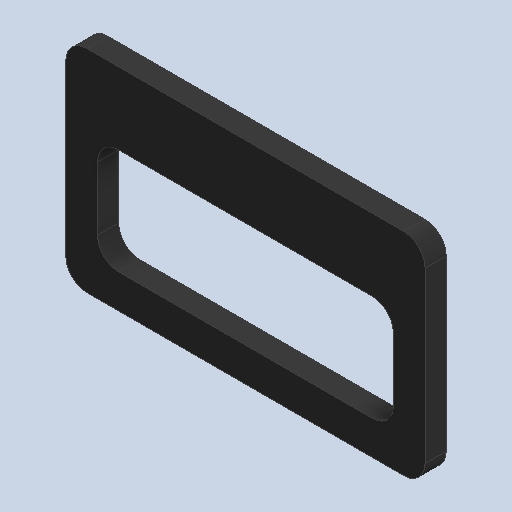
# Autodesk Inventor part: CAMERA_CON_SPACER
Saved by Autodesk Inventor 2024.2 (Build 282272000, 272)
## iProperties
Created: 2020-06-21
Part Number: CAMERA_CON_SPACER
Material: Generic
Document SubType Name: Modeling
Designer: Viktor Lindström
Density: 1 g/cm^3
Appearance: Default
Author: Viktor Lindström
Autodesk Inventor part; units mm, degrees
ref_plane "YZ Plane" through (0, 0, 0) normal (1, 0, 0) x (0, 1, 0)
ref_plane "XZ Plane" through (0, 0, 0) normal (0, 1, 0) x (-1, 0, 0)
ref_plane "XY Plane" through (0, 0, 0) normal (0, 0, 1) x (1, 0, 0)
sketch "Sketch1" plane through (0, 0, 0) normal (0, 0, 1) x (1, 0, 0)
  line L0 (-8.5, -5) -> (8.5, -5)
  line L1 (8.5, -5) -> (8.5, 5)
  line L2 (8.5, 5) -> (-8.5, 5)
  line L3 (-8.5, 5) -> (-8.5, -5)
  line L4 (-8.5, -5) -> (8.5, 5) construction
  line L5 (8.5, -5) -> (-8.5, 5) construction
  line L6 (0, -7) -> (0, 7) construction
  line L7 (-7, -3.4) -> (7, -3.4)
  line L8 (7, -3.4) -> (7, 1.6)
  line L9 (7, 1.6) -> (-7, 1.6)
  line L10 (-7, 1.6) -> (-7, -3.4)
  line L11 (-7, -3.4) -> (7, 1.6) construction
  line L12 (7, -3.4) -> (-7, 1.6) construction
  point P0 (0, 0)
  point P1 (0, -0.9)
  dimension "d0" = 10
  dimension "d1" = 17
  dimension "d2" = 4.1
  dimension "d3" = 5
  dimension "d4" = 14
  constraints: 24 end point, 4 midpoint, 4 parallel, 2 horizontal, 2 perpendicular, 1 point on line
  measures "d0" distance of L2.end L0.start
  measures "d1" distance of L1.end L2.end
  measures "d2" distance from line of L0 point (0, -0.9)
  measures "d3" distance between parallel lines of L7 L9
  measures "d4" distance between parallel lines of L8 L10
extrude "Extrusion1" add sketch "Sketch1" along normal blind 1
fillet "Fillet1" radius 1 4 edges at (8.5, 5, 0.5) (8.5, -5, 0.5) (-8.5, -5, 0.5) (-8.5, 5, 0.5)
fillet "Fillet2" radius 1 4 edges at (7, 1.6, 0.5) (7, -3.4, 0.5) (-7, -3.4, 0.5) (-7, 1.6, 0.5)
body "Solid1"
